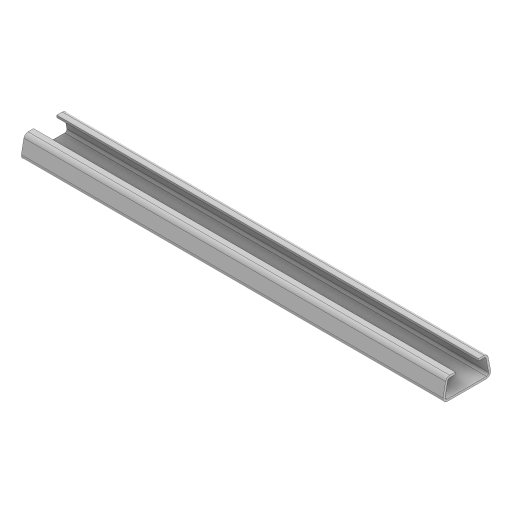
# Autodesk Inventor part: 3932-200
Saved by Autodesk Inventor 2024.3 (Build 283343000, 343)
## iProperties
Category: PARTsolutions
Company: KABELSCHLEPP
Created: 2025-09-04
Part Number: 3932-200
Material: Generic
Catalog Web Link: www.cadenas.de
Description: C-Rail-Assembly profile bars for strain relief devices
Vendor: KABELSCHLEPP
Document SubType Name: Modeling
Designer: psAdmin
Manufacturer: KABELSCHLEPP
Mass: 82.1383 g
Surface Area: 482.566 cm^2
Volume: 82.1383 cm^3
Density: 1 g/cm^3
Appearance: PSOLRGB-175-175-175
PSOL_IDENT_0: {$CADENAS_DATA/23d-libs/kabelschlepp/zubehoer/c_schiene.prj},158 {VTYP=3D},{NB=3932-200},{LINA=3932-
PSOL_IDENT_1: 200},{NN=C-Rail},{DATE=04.04.2025 14:48:42},{GEOMDATE=04.04.2025 12:06:56},{VERSION=},{LINEID=50},{W
PSOL_IDENT_2: BVAR=L},{WBNUMERIC=L}  {NB=3932-200},{LINA=3932-200},{KT=DUMMY},{CNSORDERNO=3932-200},{ARTNR=3932},{
PSOL_IDENT_3: BEZ=C-Schiene 34 x 15 mm},{CNSMAT=Stahl},{L=200},{LALG=200,[1:3000]},{INFO=PDF Katalog},{VERS=4}
NB: 3932-200
NN: C-Rail
NT: Assembly profile bars for strain relief devices
NBSYN: $ARTNR.-$L.
LINA: 3932-200
CATALOG: Kabelschlepp
CNSORDERNO: 3932-200
ARTNR: 3932
BEZ: C-Rail 34 x 15 mm
CNSMAT: Steel
L: 200
SUPPLIER: KABELSCHLEPP
ARTICLENO: 3932-200
BOMINFO: 3932-200
CREATOR: CADENAS GmbH
Title: 3932-200
Author: Cadenas PARTsolutions
Comments: Assembly profile bars for strain relief devices
Autodesk Inventor part; units mm, degrees
ref_plane "S1_XY" through (0, -1.5, 0) normal (-1, 0, 0) x (0, 0, -1)
ref_plane "S1_YZ" through (0, -1.5, 0) normal (0, 0, -1) x (0, -1, 0)
ref_plane "S1_ZX" through (0, -1.5, 0) normal (0, -1, 0) x (-1, 0, 0)
ref_plane "S2_XY" through (200, -1.5, 0) normal (1, 0, 0) x (0, 0, -1)
ref_plane "S2_YZ" through (200, -1.5, 0) normal (0, 0, -1) x (0, 1, 0)
ref_plane "S2_ZX" through (200, -1.5, 0) normal (0, 1, 0) x (1, 0, 0)
sketch "Sketch_1" plane through (0, 0, 0) normal (1, 0, 0) x (0, 1, 0)
  arc A0 (2.073, 16.9448) -> (-1.5, 14) centre (1.5, 14) ccw
  line L0 (-1.5, 14) -> (-1.5, -14)
  arc A1 (-1.5, -14) -> (2.073, -16.9448) centre (1.5, -14) ccw
  line L1 (2.073, -16.9448) -> (11.373, -15.1352)
  arc A2 (11.373, -15.1352) -> (13.8, -12.1904) centre (10.8, -12.1904) ccw
  line L2 (13.8, -12.1904) -> (13.8, -8.25)
  line L3 (13.8, -8.25) -> (12.3, -8.25)
  line L4 (12.3, -8.25) -> (12.3, -12.1904)
  arc A3 (11.0865, -13.6628) -> (12.3, -12.1904) centre (10.8, -12.1904) ccw
  line L5 (11.0865, -13.6628) -> (1.7865, -15.4724)
  arc A4 (0, -14) -> (1.7865, -15.4724) centre (1.5, -14) ccw
  line L6 (0, -14) -> (0, 14)
  arc A5 (1.7865, 15.4724) -> (0, 14) centre (1.5, 14) ccw
  line L7 (1.7865, 15.4724) -> (11.0865, 13.6628)
  arc A6 (12.3, 12.1904) -> (11.0865, 13.6628) centre (10.8, 12.1904) ccw
  line L8 (12.3, 12.1904) -> (12.3, 8.25)
  line L9 (12.3, 8.25) -> (13.8, 8.25)
  line L10 (13.8, 8.25) -> (13.8, 12.1904)
  arc A7 (13.8, 12.1904) -> (11.373, 15.1352) centre (10.8, 12.1904) ccw
  line L11 (11.373, 15.1352) -> (2.073, 16.9448)
  constraints: 24 end point, 16 point on circle, 8 centre point
extrude "Extrusion1" add sketch "Sketch_1" along normal blind 200 and the other way blind 100
sketch "Sketch2" plane through (-100, -1.5, -14) normal (0, -1, 0) x (1, 0, 0)
  circle A0 centre (26.56, 10.8287) radius 19.7262
  point P0 (100, 14)
  constraints: 1 centre point
sketch "草图3" plane through (200, -1.5, -14) normal (0, -1, 0) x (1, 0, 0)
  circle A0 centre (-27.2013, 14) radius 12.4918
  point P0 (-200, 14)
  constraints: 1 centre point
sketch "草图4" plane through (-100, 0, 0) normal (-1, 0, 0) x (0, 0, 1)
  circle A0 centre (11.9436, 5.123) radius 5.6638
  point P0 (0, 0)
  constraints: 1 centre point
body "Solid1"
